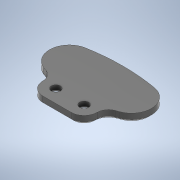
# Autodesk Inventor part: 08-04-01-006_clutchPlateRight
Saved by Autodesk Inventor 2020 (Build 240168000, 168)
## iProperties
Created: 2021-08-01
Part Number: 08-04-01-006_clutchPlateRight
Material: ABS-Kunststoff(1)
Document SubType Name: Modeling
Designer: Eric
Density: 1.06 g/cm^3
Appearance: Glatt - Weiß(1)
Mass: 1.39589 g
Surface Area: 11.6325 cm^2
Volume: 1.31688 cm^3
Author: Eric
## iProperties of the stored document _3D-Druck.ipt
Created: 2021-08-29
Part Number: _3D-Druck
Material: Generisch
Document SubType Name: Modeling
Designer: Eric
Density: 1 g/cm^3
Appearance: Vorgabe
Author: Eric
Autodesk Inventor part; units mm, degrees
ref_plane "YZ Plane" through (0, 0, 0) normal (1, 0, 0) x (0, 1, 0)
ref_plane "XZ Plane" through (0, 0, 0) normal (0, 1, 0) x (-1, 0, 0)
ref_plane "XY Plane" through (0, 0, 0) normal (0, 0, 1) x (1, 0, 0)
sketch "Skizze1" plane through (0, 0, 0) normal (0, 1, 0) x (-1, 0, 0)
  circle A0 centre (0, 0) radius 1.6
  circle A1 centre (-10, 0) radius 1.6
  line L0 (0, 4.6) -> (-10, 4.6)
  arc A2 (-10, 4.6) -> (-14.6, 0) centre (-10, 0) ccw
  arc A3 (-17.2319, -3.7588) -> (-14.6, 0) centre (-18.6, 0) ccw
  arc A4 (4.6, 0) -> (0, 4.6) centre (0, 0) ccw
  arc A5 (4.6, 0) -> (7.2319, -3.7588) centre (8.6, 0) ccw
  line L1 (7.2319, -3.7588) -> (8.3941, -4.1818)
  arc A6 (7.2222, -17.6521) -> (8.3941, -4.1818) centre (6, -10.7596) ccw
  arc A7 (-17.2222, -17.6521) -> (7.2222, -17.6521) centre (-5, 51.2726) ccw
  line L2 (-17.2319, -3.7588) -> (-18.3941, -4.1818)
  arc A8 (-18.3941, -4.1818) -> (-17.2222, -17.6521) centre (-16, -10.7596) ccw
  dimension "d0" = 10
  dimension "d1" = 3.2
  dimension "d2" = 3
  dimension "d4" = 4
  dimension "d22" = 7
  dimension "d23" = 20
  dimension "d24" = 22
  dimension "d25" = 70
  constraints: 14 point on circle, 10 tangent, 9 centre point, 6 end point, 4 horizontal alignment, 3 equal radius, 2 concentric, 1 coincident, 1 equal length, 1 horizontal
  measures "d0" distance of point (0, 0) A1.centre
  measures "d1" diameter of A0
  measures "d2" radial gap between concentric circles of A0 A4
  measures "d4" radius of A3
  measures "d22" radius of A8
  measures "d23" angle of L0 L2
  measures "d24" distance of A6.centre A8.centre
  measures "d25" radius of A7
extrude "Extrusion1" add sketch "Skizze1" along normal blind 3
chamfer "Fase1" distance 1 angle 45 10 edges at (13.2527, 0, 3.2527) (15.3234, 0, -2.2943) (17.813, 0, -3.9703) (22.9737, 0, -11.3663) (5, 0, -18.7274) (-12.9737, 0, -11.3663) (-7.813, 0, -3.9703) (-5.3234, 0, -2.2943) (-3.2527, 0, 3.2527) (5, 0, 4.6)
chamfer "Fase3" distance 1.5 angle 45 2 edges at (11.6, 0, 0) (1.6, 0, 0)
